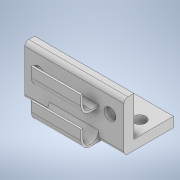
# Autodesk Inventor part: giá đỡ vòi
Saved by Autodesk Inventor 2020 (Build 240168000, 168)
## iProperties
Created: 2022-09-22
Part Number: giá đỡ vòi
Material: Generic
Document SubType Name: Modeling
Designer: ASUS
Density: 1 g/cm^3
Appearance: Default
Author: ASUS
Autodesk Inventor part; units mm, degrees
ref_plane "YZ Plane" through (0, 0, 0) normal (1, 0, 0) x (0, 1, 0)
ref_plane "XZ Plane" through (0, 0, 0) normal (0, 1, 0) x (-1, 0, 0)
ref_plane "XY Plane" through (0, 0, 0) normal (0, 0, 1) x (1, 0, 0)
sketch "Sketch1" plane through (0, 0, 0) normal (0, 0, 1) x (1, 0, 0)
  line L0 (0, 0) -> (25, 0)
  line L1 (25, 0) -> (25, 25)
  line L2 (25, 25) -> (0, 25)
  line L3 (0, 25) -> (0, 0)
  dimension "d0" = 25
  dimension "d1" = 25
  constraints: 8 end point, 2 parallel, 1 horizontal, 1 perpendicular
  measures "d0" distance of L2.end L1.end
  measures "d1" distance of L1.end L0.end
extrude "Extrusion1" add sketch "Sketch1" along normal blind 5
sketch "Sketch2" plane through (0, 0, 0) normal (0, 0, -1) x (-1, 0, 0)
  line L0 (0, 25) -> (0, 0) projected
  line L1 (-25, 0) -> (-25, 25) projected
  line L2 (0, 0) -> (-25, 0)
  line L3 (-25, 0) -> (-25, 5)
  line L4 (-25, 5) -> (0, 5)
  line L5 (0, 5) -> (0, 0)
  dimension "d4" = 5
  constraints: 8 end point, 2 parallel, 1 horizontal, 1 perpendicular, 1 point on line
  measures "d4" distance of L2.end L3.end
extrude "Extrusion2" add sketch "Sketch2" along normal blind 20
sketch "Sketch3" plane through (0, 5, 0) normal (0, 1, 0) x (1, 0, 0)
  circle A0 centre (7, 10) radius 3
  line L0 (0, 20) -> (25, 20) projected
  line L1 (0, 0) -> (0, 20) projected
  dimension "d8" = 6
  dimension "d13" = 10
  dimension "d19" = 7
  constraints: 1 centre point
  measures "d8" diameter of A0
  measures "d13" distance from line of L0 A0.centre
  measures "d19" distance from line of L1 A0.centre
extrude "Extrusion3" cut sketch "Sketch3" against normal through all
sketch "Sketch4" plane through (0, 0, 0) normal (0, 0, -1) x (-1, 0, 0)
  circle A0 centre (-7, 15) radius 3
  line L0 (-25, 25) -> (0, 25) projected
  line L1 (0, 25) -> (0, 5) projected
  point P0 (0, 0)
  dimension "d11" = 6
  dimension "d12" = 10
  dimension "d20" = 7
  constraints: 1 centre point
  measures "d11" diameter of A0
  measures "d12" distance from line of L0 A0.centre
  measures "d20" distance from line of L1 A0.centre
extrude "Extrusion4" cut sketch "Sketch4" against normal through all
move faces "Move1" translate (25, 0, 0) faces at (25, 10, 3.3333)
sketch "Sketch5" plane through (0, 5, 0) normal (0, 1, 0) x (1, 0, 0)
  circle A0 centre (43, 10) radius 3
  line L0 (50, 0) -> (50, 20) projected
  point P0 (0, 0)
  dimension "d21" = 6
  dimension "d22" = 7
  constraints: 1 centre point
  measures "d21" diameter of A0
  measures "d22" distance from line of L0 A0.centre
extrude "Extrusion5" cut sketch "Sketch5" against normal through all
sketch "Sketch6" plane through (0, 0, 0) normal (0, 0, -1) x (-1, 0, 0)
  circle A0 centre (-43, 15) radius 3
  line L0 (-50, 5) -> (-50, 25) projected
  point P0 (0, 0)
  dimension "d25" = 6
  dimension "d26" = 7
  constraints: 1 centre point
  measures "d25" diameter of A0
  measures "d26" distance from line of L0 A0.centre
extrude "Extrusion6" cut sketch "Sketch6" against normal through all
sketch "Sketch7" plane through (0, 0, 5) normal (0, 0, 1) x (1, 0, 0)
  line L0 (50, 25) -> (0, 25) projected
  line L1 (50, 0) -> (0, 0) projected
  line L2 (12.3464, 25) -> (37.3464, 25)
  line L3 (37.3464, 25) -> (37.3464, 0)
  line L4 (37.3464, 0) -> (12.3464, 0)
  line L5 (12.3464, 0) -> (12.3464, 25)
  dimension "d29" = 25
  constraints: 8 end point, 2 parallel, 2 point on line, 1 horizontal, 1 perpendicular
  measures "d29" distance of L3.end L4.end
extrude "Extrusion7" add sketch "Sketch7" along normal blind 10
ref_plane "Work Plane1" through (37.3464, 0, 5) normal (1, 0, 0) x (0, 0, -1)
sketch "Sketch8" plane through (37.3464, 0, 5) normal (1, 0, 0) x (0, 0, -1)
  line L0 (0, 25) -> (-10, 25) projected
  line L1 (-10, 20) -> (-10, 10)
  line L2 (0, 10) -> (0, 20)
  line L3 (0, 25) -> (0, 0) projected
  line L4 (0, 10) -> (0, 18) projected
  line L5 (0, 10) -> (0, 20)
  line L6 (0, 20) -> (0, 10)
  line L7 (0, 0) -> (-10, 0) projected
  line L8 (0, 25) -> (0, 0) projected
  arc A0 (-8, 20) -> (-4, 16) centre (-4, 20) ccw
  line L9 (-4, 16) -> (0, 16)
  line L10 (-8, 20) -> (-2.9809, 20) construction
  arc A1 (-8, 5) -> (0, 5) centre (-4, 5) ccw
  arc A2 (-9, 5) -> (0, 8) centre (-4, 5) ccw
  line L11 (-10, 10) -> (0, 10)
  line L12 (-10, 25) -> (-10, 0) projected
  line L13 (-9.4374, 25) -> (0, 25)
  line L14 (0, 17) -> (0, 25)
  line L15 (-4, 15) -> (0, 15)
  arc A3 (0, 17) -> (0, 23) centre (-4, 20) ccw
  arc A4 (-9, 20) -> (-4, 15) centre (-4, 20) ccw
  line L16 (-10.1199, 0) -> (-4, 0)
  line L17 (-8, 5) -> (-2.9809, 5) construction
  line L18 (-10, 10) -> (-10, 0)
  line L19 (-10, 0) -> (-4, 0)
  line L20 (-9, 5) -> (-9.1746, 10)
  line L21 (-9, 5) -> (-3.997, 5) construction
  line L22 (-8, 5) -> (-8.1746, 10)
  line L23 (-8, 5) -> (-2.997, 5) construction
  line L24 (-9, 20) -> (-9.1746, 25)
  line L25 (0, 25) -> (-10, 25) projected
  line L26 (-9, 20) -> (-3.997, 20) construction
  line L27 (-8, 20) -> (-8.1746, 25)
  line L28 (-8, 20) -> (-2.997, 20) construction
  point P0 (5, 0)
  point P1 (-10, 12)
  point P2 (0, 5)
  point P3 (-9.1746, 25)
  dimension "d60" = 8
  dimension "d61" = 4
  dimension "d62" = 5
  dimension "d64" = 8
  dimension "d65" = 4
  dimension "d66" = 5
  dimension "d70" = 92
  dimension "d71" = 92
  dimension "d72" = 92
  dimension "d73" = 92
  constraints: 44 end point, 11 point on circle, 8 point on line, 7 horizontal, 5 centre point, 4 collinear, 4 equal length, 3 tangent, 2 coincident, 2 perpendicular, 1 vertical, 7 other
  measures "d60" diameter of A0
  measures "d61" distance from line of L3 A0.centre
  measures "d62" distance from line of L0 A0.centre
  measures "d64" diameter of A1
  measures "d65" distance from line of L3 A1.centre
  measures "d66" distance from line of L7 A1.centre
  measures "d70" angle of L21 L20
  measures "d71" angle of L23 L22
  measures "d72" angle of L26 L24
  measures "d73" angle of L28 L27
extrude "Extrusion13" cut sketch "Sketch8" against normal through all contours L3 L2 L9 A0 L27 L0 | L24 A4 L15 L2 L11 L1 L12 L0 | L3 A1 L22 L11 | L11 L20 A2 L7 L12
fillet "Fillet3" radius 2 3 edges at (43.6732, 0, 5) (6.1732, 0, 5) (25, 25, 5)
body "Solid1"
